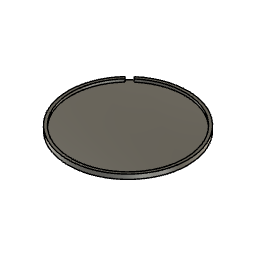
MedWise_lid v1 (Autodesk Fusion 360 design; units mm, degrees)
Autodesk Fusion 360 part; units mm, degrees
note: some values were not read from the file. Set by a fixed rule: which sketch regions a step uses.
sketch "Sketch1" plane through (0, 0, 0) normal (0, 0, 1) x (1, 0, 0)
  circle A0 centre (0, 0) radius 65
  dimension "d1" = 130
  constraint coincident A0.centre origin
  measures "d1" diameter of A0
extrude "Extrude1" add sketch "Sketch1" along normal blind 5
hole "Hole1" at (0, 0, 5) direction (0, 0, -1) diameter 124 depth 3 tip angle 180
sketch "Sketch2" plane through (0, 0, 5) normal (0, 0, 1) x (-1, 0, 0)
  circle A0 centre (0, 0) radius 62
  circle A1 centre (0, 0) radius 65
  line L0 (54.116, -50.8938) -> (49.1662, -55.8435)
  line L1 (49.1662, -55.8435) -> (34.7966, -41.4739)
  line L2 (34.7966, -41.4739) -> (39.7463, -36.5241)
  line L3 (39.7463, -36.5241) -> (54.116, -50.8938)
  dimension "d7" = 7
  constraint perpendicular L0 L1
  constraint parallel L0 L2
  constraint parallel L1 L3
  measures "d7" distance of L0.start L0.end
extrude "Extrude2" cut sketch "Sketch2" against normal blind 3 contours A0 A1 L1 L3 picked at (41.6647, -47.2432)
